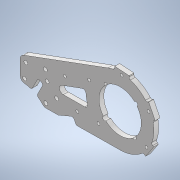
# Autodesk Inventor part: motor_h_6
Saved by Autodesk Inventor 2020 (Build 240168000, 168)
## iProperties
Created: 2020-11-16
Part Number: motor_h_6
Material: Generic
Document SubType Name: Modeling
Designer: Shuang Peng
Density: 1 g/cm^3
Appearance: Default
Author: Shuang Peng
Autodesk Inventor part; units mm, degrees
ref_plane "YZ Plane" through (0, 0, 0) normal (1, 0, 0) x (0, 1, 0)
ref_plane "XZ Plane" through (0, 0, 0) normal (0, 1, 0) x (-1, 0, 0)
ref_plane "XY Plane" through (0, 0, 0) normal (0, 0, 1) x (1, 0, 0)
sketch "Sketch1" plane through (0, 0, 0) normal (0, 0, 1) x (1, 0, 0)
  circle A0 centre (0.5323, 0.2768) radius 22 projected
  circle A1 centre (0.5323, 0.2768) radius 35
  line L0 (-78.3162, -45.1599) -> (-53.6214, -37.0254) projected
  line L1 (-86.2398, -25.4424) -> (-79.6785, -13.735) projected
  line L2 (-88.6848, -24.2091) -> (-83.1688, -11.9743) projected
  line L3 (-114.2243, 0.9226) -> (-109.1572, -20.6268) projected
  circle A2 centre (-76.7687, -31.0745) radius 2 projected
  circle A3 centre (-65.488, -21.1879) radius 2 projected
  circle A4 centre (-98.8432, -19.9393) radius 2 projected
  circle A5 centre (-97.5964, -4.9912) radius 2 projected
  line L4 (-9.6196, 33.6521) -> (-104.4582, 6.5421) projected
  line L5 (-65.488, -21.1879) -> (-97.5964, -4.9912)
  line L6 (-97.5964, -4.9912) -> (-98.8432, -19.9393)
  line L7 (-98.8432, -19.9393) -> (-76.7687, -31.0745)
  line L8 (-76.7687, -31.0745) -> (-65.488, -21.1879)
  arc A6 (-123.4396, -70.4026) -> (-119.9166, -61.7947) centre (-170.0752, -46.291) ccw projected
  arc A7 (-116.2774, -61.379) -> (-119.9166, -61.7947) centre (-118.0058, -62.3853) ccw projected
  arc A8 (-116.2774, -61.379) -> (-113.2569, -65.1861) centre (-101.5862, -52.8251) ccw projected
  arc A9 (-113.5219, -68.3053) -> (-113.2569, -65.1861) centre (-114.63, -66.6404) ccw projected
  line L9 (-113.5219, -68.3053) -> (-120.5549, -72.9861) projected
  arc A10 (-123.4396, -70.4026) -> (-120.5549, -72.9861) centre (-121.663, -71.3211) ccw projected
  arc A11 (-108.797, -37.4302) -> (-114.395, -41.6477) centre (-101.5862, -52.8251) ccw projected
  arc A12 (-117.8899, -40.5514) -> (-114.395, -41.6477) centre (-115.9019, -40.3327) ccw projected
  arc A13 (-117.8899, -40.5514) -> (-120.2217, -29.8328) centre (-170.0752, -46.291) ccw projected
  arc A14 (-117.1337, -27.5974) -> (-120.2217, -29.8328) centre (-118.3225, -29.2058) ccw projected
  line L10 (-117.1337, -27.5974) -> (-108.4566, -34.0106) projected
  arc A15 (-108.797, -37.4302) -> (-108.4566, -34.0106) centre (-109.6453, -35.619) ccw projected
  circle A16 centre (-99.5268, -40.1525) radius 2.05 projected
  circle A17 centre (-114.2588, -50.7657) radius 2.05 projected
  circle A18 centre (-103.6456, -65.4977) radius 2.05 projected
  circle A19 centre (-88.9136, -54.8845) radius 2.05 projected
  circle A20 centre (-108.8928, -42.6829) radius 1.55 projected
  circle A21 centre (-94.2796, -62.9673) radius 1.55 projected
  circle A22 centre (-111.7284, -60.1317) radius 1.55 projected
  circle A23 centre (-91.444, -45.5185) radius 1.55 projected
  line L11 (-163.6957, -101.6981) -> (-176.5687, -110.2656) projected
  arc A24 (-179.6679, -108.4127) -> (-176.5687, -110.2656) centre (-177.6768, -108.6006) ccw projected
  arc A25 (-179.6679, -108.4127) -> (-179.6132, -104.4918) centre (-204.0596, -106.1116) ccw projected
  arc A26 (-178.2819, -101.796) -> (-179.6132, -104.4918) centre (-176.6198, -104.2934) ccw projected
  line L12 (-178.2819, -101.796) -> (-174.2482, -99.1114) projected
  arc A27 (-171.3549, -98.2753) -> (-174.2482, -99.1114) centre (-171.4779, -103.2738) ccw projected
  arc A28 (-171.3549, -98.2753) -> (-164.9991, -98.0427) centre (-170.0752, -46.291) ccw projected
  arc A29 (-163.6957, -101.6981) -> (-164.9991, -98.0427) centre (-164.8038, -100.0331) ccw projected
  arc A30 (-215.7892, -71.0747) -> (-212.0199, -77.0261) centre (-170.0752, -46.291) ccw projected
  arc A31 (-212.9841, -80.1) -> (-212.0199, -77.0261) centre (-213.6331, -78.2082) ccw projected
  arc A32 (-212.9841, -80.1) -> (-217.4538, -82.094) centre (-204.0596, -106.1116) ccw projected
  arc A33 (-220.4168, -80.1368) -> (-217.4538, -82.094) centre (-218.4279, -80.3472) ccw projected
  line L13 (-220.4168, -80.1368) -> (-219.5364, -71.8174) projected
  arc A34 (-215.7892, -71.0747) -> (-219.5364, -71.8174) centre (-217.5475, -72.0279) ccw projected
  circle A35 centre (-195.3093, -126.2965) radius 2.05 projected
  circle A36 centre (-183.8747, -97.3613) radius 2.05 projected
  circle A37 centre (-212.81, -85.9267) radius 2.05 projected
  circle A38 centre (-224.2445, -114.862) radius 2.05 projected
  circle A39 centre (-156.8228, -41.9256) radius 2.1 projected
  circle A40 centre (-142.9852, -15.9584) radius 2.1 projected
  circle A41 centre (-167.2295, -32.6314) radius 2.1 projected
  circle A42 centre (-182.799, -7.6641) radius 2.1 projected
  circle A43 centre (-180.482, -36.9968) radius 2.1 projected
  circle A44 centre (-209.889, -37.9967) radius 2.1 projected
  circle A45 centre (-183.3277, -50.6564) radius 2.1 projected
  circle A46 centre (-197.1652, -76.6237) radius 2.1 projected
  circle A47 centre (-172.9209, -59.9507) radius 2.1 projected
  circle A48 centre (-157.3514, -84.918) radius 2.1 projected
  circle A49 centre (-130.2614, -54.5854) radius 2.1 projected
  circle A50 centre (-159.6685, -55.5853) radius 2.1 projected
  line L14 (-151.4769, -35.1571) -> (-159.0568, -36.2537) projected
  arc A51 (-161.3422, -34.2126) -> (-159.0568, -36.2537) centre (-159.3431, -34.2743) ccw projected
  line L15 (-161.3422, -34.2126) -> (-161.1059, -26.5575) projected
  arc A52 (-156.5463, -24.0882) -> (-161.1059, -26.5575) centre (-158.1073, -26.65) ccw projected
  arc A53 (-149.5366, -30.3485) -> (-156.5463, -24.0882) centre (-170.0752, -46.291) ccw projected
  arc A54 (-151.4769, -35.1571) -> (-149.5366, -30.3485) centre (-151.9064, -32.188) ccw projected
  line L16 (-170.4183, -24.6174) -> (-173.2586, -31.7301) projected
  arc A55 (-176.1689, -32.6888) -> (-173.2586, -31.7301) centre (-175.1159, -30.9884) ccw projected
  line L17 (-176.1689, -32.6888) -> (-182.6803, -28.6566) projected
  arc A56 (-182.539, -23.4732) -> (-182.6803, -28.6566) centre (-181.1009, -26.106) ccw projected
  arc A57 (-173.6125, -20.5328) -> (-182.539, -23.4732) centre (-170.0752, -46.291) ccw projected
  arc A58 (-170.4183, -24.6174) -> (-173.6125, -20.5328) centre (-173.2044, -23.5049) ccw projected
  line L18 (-189.0166, -35.7513) -> (-184.277, -41.7674) projected
  arc A59 (-184.9019, -44.7672) -> (-184.277, -41.7674) centre (-185.848, -43.0051) ccw projected
  line L19 (-184.9019, -44.7672) -> (-191.6497, -48.3902) projected
  arc A60 (-196.0679, -45.6761) -> (-191.6497, -48.3902) centre (-193.0688, -45.747) ccw projected
  arc A61 (-194.1512, -36.4753) -> (-196.0679, -45.6761) centre (-170.0752, -46.291) ccw projected
  arc A62 (-189.0166, -35.7513) -> (-194.1512, -36.4753) centre (-191.3732, -37.6079) ccw projected
  line L20 (-188.6736, -57.4249) -> (-181.0937, -56.3283) projected
  arc A63 (-178.8083, -58.3694) -> (-181.0937, -56.3283) centre (-180.8073, -58.3077) ccw projected
  line L21 (-178.8083, -58.3694) -> (-179.0445, -66.0246) projected
  arc A64 (-183.6042, -68.4939) -> (-179.0445, -66.0246) centre (-182.0431, -65.932) ccw projected
  arc A65 (-190.6139, -62.2336) -> (-183.6042, -68.4939) centre (-170.0752, -46.291) ccw projected
  arc A66 (-188.6736, -57.4249) -> (-190.6139, -62.2336) centre (-188.244, -60.394) ccw projected
  line L22 (-169.7321, -67.9646) -> (-166.8919, -60.8519) projected
  arc A67 (-163.9815, -59.8933) -> (-166.8919, -60.8519) centre (-165.0345, -61.5936) ccw projected
  line L23 (-163.9815, -59.8933) -> (-157.4701, -63.9255) projected
  arc A68 (-157.6114, -69.1089) -> (-157.4701, -63.9255) centre (-159.0496, -66.4761) ccw projected
  arc A69 (-166.5379, -72.0493) -> (-157.6114, -69.1089) centre (-170.0752, -46.291) ccw projected
  arc A70 (-169.7321, -67.9646) -> (-166.5379, -72.0493) centre (-166.9461, -69.0772) ccw projected
  line L24 (-151.1338, -56.8307) -> (-155.8734, -50.8146) projected
  arc A71 (-155.2485, -47.8149) -> (-155.8734, -50.8146) centre (-154.3024, -49.5769) ccw projected
  line L25 (-155.2485, -47.8149) -> (-148.5008, -44.1919) projected
  arc A72 (-144.0825, -46.906) -> (-148.5008, -44.1919) centre (-147.0817, -46.835) ccw projected
  arc A73 (-145.9993, -56.1068) -> (-144.0825, -46.906) centre (-170.0752, -46.291) ccw projected
  arc A74 (-151.1338, -56.8307) -> (-145.9993, -56.1068) centre (-148.7773, -54.9742) ccw projected
  arc A75 (-216.0243, -48.4556) -> (-208.3152, -71.8586) centre (-170.0752, -46.291) ccw projected
  arc A76 (-211.8355, -44.272) -> (-216.0243, -48.4556) centre (-212.0287, -48.2673) ccw projected
  line L26 (-211.8355, -44.272) -> (-205.407, -44.5828) projected
  arc A77 (-202.5538, -47.4705) -> (-205.407, -44.5828) centre (-205.5518, -47.5793) ccw projected
  arc A78 (-202.5538, -47.4705) -> (-196.8964, -64.6451) centre (-170.0752, -46.291) ccw projected
  arc A79 (-197.4748, -68.6631) -> (-196.8964, -64.6451) centre (-199.3722, -66.3394) ccw projected
  line L27 (-197.4748, -68.6631) -> (-202.4602, -72.7337) projected
  arc A80 (-208.3152, -71.8586) -> (-202.4602, -72.7337) centre (-204.99, -69.6353) ccw projected
  arc A81 (-191.1752, -87.1663) -> (-167.0531, -92.1917) centre (-170.0752, -46.291) ccw projected
  arc A82 (-192.7039, -81.447) -> (-191.1752, -87.1663) centre (-189.3404, -83.612) ccw projected
  line L28 (-192.7039, -81.447) -> (-189.2204, -76.0351) projected
  arc A83 (-185.2931, -75.008) -> (-189.2204, -76.0351) centre (-186.6978, -77.6588) ccw projected
  arc A84 (-185.2931, -75.008) -> (-167.5907, -78.6959) centre (-170.0752, -46.291) ccw projected
  arc A85 (-164.4002, -81.2059) -> (-167.5907, -78.6959) centre (-167.3614, -81.6872) ccw projected
  line L29 (-164.4002, -81.2059) -> (-163.3677, -87.5586) projected
  arc A86 (-167.0531, -92.1917) -> (-163.3677, -87.5586) centre (-167.3159, -88.2003) ccw projected
  arc A87 (-145.2262, -85.0018) -> (-128.813, -66.6241) centre (-170.0752, -46.291) ccw projected
  arc A88 (-150.9436, -83.466) -> (-145.2262, -85.0018) centre (-147.3869, -81.6357) ccw projected
  line L30 (-150.9436, -83.466) -> (-153.8887, -77.7433) projected
  arc A89 (-152.8145, -73.8286) -> (-153.8887, -77.7433) centre (-151.2212, -76.3705) ccw projected
  arc A90 (-152.8145, -73.8286) -> (-140.7695, -60.3418) centre (-170.0752, -46.291) ccw projected
  arc A91 (-137.0006, -58.8338) -> (-140.7695, -60.3418) centre (-138.0644, -61.6388) ccw projected
  line L31 (-137.0006, -58.8338) -> (-130.9827, -61.1159) projected
  arc A92 (-128.813, -66.6241) -> (-130.9827, -61.1159) centre (-132.4011, -64.856) ccw projected
  arc A93 (-124.1262, -44.1265) -> (-131.8352, -20.7235) centre (-170.0752, -46.291) ccw projected
  arc A94 (-128.3149, -48.3101) -> (-124.1262, -44.1265) centre (-128.1217, -44.3147) ccw projected
  line L32 (-128.3149, -48.3101) -> (-134.7435, -47.9993) projected
  arc A95 (-137.5966, -45.1116) -> (-134.7435, -47.9993) centre (-134.5986, -45.0028) ccw projected
  arc A96 (-137.5966, -45.1116) -> (-143.254, -27.9369) centre (-170.0752, -46.291) ccw projected
  arc A97 (-142.6756, -23.9189) -> (-143.254, -27.9369) centre (-140.7782, -26.2427) ccw projected
  line L33 (-142.6756, -23.9189) -> (-137.6903, -19.8484) projected
  arc A98 (-131.8352, -20.7235) -> (-137.6903, -19.8484) centre (-135.1604, -22.9467) ccw projected
  arc A99 (-148.9752, -5.4157) -> (-173.0974, -0.3904) centre (-170.0752, -46.291) ccw projected
  arc A100 (-147.4465, -11.1351) -> (-148.9752, -5.4157) centre (-150.81, -8.9701) ccw projected
  line L34 (-147.4465, -11.1351) -> (-150.93, -16.547) projected
  arc A101 (-154.8573, -17.574) -> (-150.93, -16.547) centre (-153.4526, -14.9232) ccw projected
  arc A102 (-154.8573, -17.574) -> (-172.5597, -13.8861) centre (-170.0752, -46.291) ccw projected
  arc A103 (-175.7502, -11.3762) -> (-172.5597, -13.8861) centre (-172.7891, -10.8949) ccw projected
  line L35 (-175.7502, -11.3762) -> (-176.7828, -5.0235) projected
  arc A104 (-173.0974, -0.3904) -> (-176.7828, -5.0235) centre (-172.8346, -4.3818) ccw projected
  arc A105 (-194.9243, -7.5803) -> (-211.3374, -25.958) centre (-170.0752, -46.291) ccw projected
  arc A106 (-189.2068, -9.116) -> (-194.9243, -7.5803) centre (-192.7635, -10.9464) ccw projected
  line L36 (-189.2068, -9.116) -> (-186.2617, -14.8387) projected
  arc A107 (-187.3359, -18.7535) -> (-186.2617, -14.8387) centre (-188.9292, -16.2115) ccw projected
  arc A108 (-187.3359, -18.7535) -> (-199.3809, -32.2402) centre (-170.0752, -46.291) ccw projected
  arc A109 (-203.1498, -33.7483) -> (-199.3809, -32.2402) centre (-202.0861, -30.9432) ccw projected
  line L37 (-203.1498, -33.7483) -> (-209.1677, -31.4662) projected
  arc A110 (-211.3374, -25.958) -> (-209.1677, -31.4662) centre (-207.7494, -27.7261) ccw projected
  circle A111 centre (-204.0596, -106.1116) radius 16 projected
  circle A112 centre (-170.0752, -46.291) radius 8 projected
  circle A113 centre (-101.5862, -52.8251) radius 8 projected
  circle A114 centre (-214.7177, -133.082) radius 1.5 projected
  circle A115 centre (-219.3611, -19.837) radius 1.5 projected
  circle A116 centre (-193.5118, 4.9009) radius 1.5 projected
  circle A117 centre (-78.1429, -40.8914) radius 1.5 projected
  circle A118 centre (-111.8739, -77.0359) radius 1.5 projected
  circle A119 centre (-81.5873, -69.9144) radius 1.5 projected
  circle A120 centre (-105.9215, -26.8789) radius 1.5 projected
  circle A121 centre (-174.6475, 9.4585) radius 1.5 projected
  circle A122 centre (-207.6497, -4.3619) radius 1.5 projected
  circle A123 centre (-232.6899, -112.2194) radius 1.5 projected
  circle A124 centre (-187.3388, -130.1411) radius 1.5 projected
  line L38 (-182.2334, -121.243) -> (-118.1865, -78.6172) projected
  arc A125 (-116.0255, -78.5818) -> (-118.1865, -78.6172) centre (-117.0784, -80.2822) ccw projected
  line L39 (-116.0255, -78.5818) -> (-110.3159, -82.1175) projected
  line L40 (-110.3159, -82.1175) -> (-109.1162, -80.1802) projected
  arc A126 (-107.0138, -79.274) -> (-109.1162, -80.1802) centre (-107.4158, -81.2331) ccw projected
  arc A127 (-107.0138, -79.274) -> (-84.9408, -74.0838) centre (-101.5862, -52.8251) ccw projected
  arc A128 (-82.6548, -73.9581) -> (-84.9408, -74.0838) centre (-83.7078, -75.6585) ccw projected
  line L41 (-82.6548, -73.9581) -> (-80.7175, -75.1578) projected
  line L42 (-80.7175, -75.1578) -> (-76.5057, -68.3563) projected
  line L43 (-76.5057, -68.3563) -> (-80.8261, -65.6809) projected
  arc A129 (-81.5538, -63.0698) -> (-80.8261, -65.6809) centre (-79.7732, -63.9805) ccw projected
  arc A130 (-81.5538, -63.0698) -> (-79.7124, -47.5537) centre (-101.5862, -52.8251) ccw projected
  arc A131 (-78.3938, -45.1855) -> (-79.7124, -47.5537) centre (-77.7681, -47.0851) ccw projected
  line L44 (-78.3938, -45.1855) -> (-73.5672, -43.5956) projected
  line L45 (-73.5672, -43.5956) -> (-76.0701, -35.9972) projected
  line L46 (-76.0701, -35.9972) -> (-78.2344, -36.7101) projected
  arc A132 (-80.4274, -36.0529) -> (-78.2344, -36.7101) centre (-78.8601, -34.8105) ccw projected
  arc A133 (-80.4274, -36.0529) -> (-100.6725, -25.8406) centre (-101.5862, -52.8251) ccw projected
  arc A134 (-102.5044, -24.4675) -> (-100.6725, -25.8406) centre (-100.6048, -23.8417) ccw projected
  line L47 (-102.5044, -24.4675) -> (-103.2174, -22.3032) projected
  line L48 (-103.2174, -22.3032) -> (-109.8332, -24.4825) projected
  arc A135 (-111.6477, -24.1912) -> (-109.8332, -24.4825) centre (-110.4589, -22.5829) ccw projected
  line L49 (-111.6477, -24.1912) -> (-138.8709, -4.0709) projected
  arc A136 (-138.8709, -4.0709) -> (-157.489, 4.6779) centre (-170.0752, -46.291) ccw projected
  arc A137 (-158.9675, 7.0275) -> (-157.489, 4.6779) centre (-157.0095, 6.6196) ccw projected
  line L50 (-158.9675, 7.0275) -> (-157.9255, 12.0294) projected
  line L51 (-157.9255, 12.0294) -> (-173.905, 13.0221) projected
  arc A138 (-173.905, 13.0221) -> (-179.0599, 12.4626) centre (-170.0752, -46.291) ccw projected
  line L52 (-179.0599, 12.4626) -> (-178.9132, 11.5029) projected
  arc A139 (-180.5204, 9.2351) -> (-178.9132, 11.5029) centre (-180.8902, 11.2006) ccw projected
  arc A140 (-180.5204, 9.2351) -> (-188.9488, 6.9634) centre (-170.0752, -46.291) ccw projected
  arc A141 (-191.4781, 8.1164) -> (-188.9488, 6.9634) centre (-189.6169, 8.8485) ccw projected
  line L53 (-191.4781, 8.1164) -> (-191.9672, 9.3596) projected
  arc A142 (-191.9672, 9.3596) -> (-197.6643, 6.7664) centre (-170.0752, -46.291) ccw projected
  line L54 (-197.6643, 6.7664) -> (-207.7018, 0.19) projected
  arc A143 (-207.7018, 0.19) -> (-212.3543, -3.9976) centre (-170.0752, -46.291) ccw projected
  line L55 (-212.3543, -3.9976) -> (-211.4098, -4.9425) projected
  arc A144 (-211.3627, -7.7217) -> (-211.4098, -4.9425) centre (-212.8242, -6.3564) ccw projected
  arc A145 (-211.3627, -7.7217) -> (-216.811, -14.5418) centre (-170.0752, -46.291) ccw projected
  arc A146 (-219.5321, -15.1098) -> (-216.811, -14.5418) centre (-218.4654, -13.418) ccw projected
  line L56 (-219.5321, -15.1098) -> (-220.3533, -14.592) projected
  arc A147 (-220.3533, -14.592) -> (-222.9247, -19.0947) centre (-170.0752, -46.291) ccw projected
  line L57 (-222.9247, -19.0947) -> (-228.3956, -34.1413) projected
  line L58 (-228.3956, -34.1413) -> (-223.3938, -35.1833) projected
  arc A148 (-221.8301, -37.477) -> (-223.3938, -35.1833) centre (-223.8017, -37.1413) ccw projected
  arc A149 (-221.8301, -37.477) -> (-222.2837, -40.7658) centre (-170.0752, -46.291) ccw projected
  line L59 (-222.2837, -40.7658) -> (-228.8679, -102.9811) projected
  arc A150 (-234.3963, -108.3336) -> (-228.8679, -102.9811) centre (-234.8346, -102.3497) ccw projected
  line L60 (-234.3963, -108.3336) -> (-236.9714, -108.5222) projected
  line L61 (-236.9714, -108.5222) -> (-236.5332, -114.5062) projected
  line L62 (-236.5332, -114.5062) -> (-234.3924, -116.3548) projected
  line L63 (-234.3924, -116.3548) -> (-232.2123, -116.1951) projected
  arc A151 (-230.2297, -117.3977) -> (-232.2123, -116.1951) centre (-232.0662, -118.1897) ccw projected
  arc A152 (-230.2297, -117.3977) -> (-219.5435, -130.0386) centre (-204.0596, -106.1116) ccw projected
  arc A153 (-218.77, -132.4527) -> (-219.5435, -130.0386) centre (-220.6301, -131.7177) ccw projected
  line L64 (-218.77, -132.4527) -> (-219.1728, -133.472) projected
  line L65 (-219.1728, -133.472) -> (-218.0478, -136.0671) projected
  line L66 (-218.0478, -136.0671) -> (-214.3278, -137.5372) projected
  line L67 (-214.3278, -137.5372) -> (-211.7327, -136.4122) projected
  line L68 (-211.7327, -136.4122) -> (-211.3299, -135.3929) projected
  arc A154 (-209.1151, -134.1596) -> (-211.3299, -135.3929) centre (-209.4699, -136.1279) ccw projected
  arc A155 (-209.1151, -134.1596) -> (-192.6744, -132.2387) centre (-204.0596, -106.1116) ccw projected
  arc A156 (-190.4053, -132.7163) -> (-192.6744, -132.2387) centre (-191.8754, -134.0722) ccw projected
  line L69 (-190.4053, -132.7163) -> (-188.9233, -134.3231) projected
  line L70 (-188.9233, -134.3231) -> (-186.0971, -134.4374) projected
  line L71 (-186.0971, -134.4374) -> (-181.6866, -130.3696) projected
  line L72 (-181.6866, -130.3696) -> (-183.1386, -128.7953) projected
  arc A157 (-182.2334, -121.243) -> (-183.1386, -128.7953) centre (-179.4631, -125.4054) ccw projected
  circle A158 centre (-98.8432, -19.9393) radius 4.5
  circle A159 centre (-76.7687, -31.0745) radius 4.5
  circle A160 centre (-101.5862, -52.8251) radius 28.5
  circle A161 centre (-97.5964, -4.9912) radius 6
  circle A162 centre (-65.488, -21.1879) radius 6
  arc A163 (33.1414, -11.2539) -> (34.2988, 6.971) centre (0, 0) ccw projected
  line L73 (-98.8432, -19.9393) -> (-103.3426, -20.0156)
  line L74 (-97.5964, -4.9912) -> (-103.5955, -5.0929)
  line L75 (-103.5955, -5.0929) -> (-103.3426, -20.0156)
  line L76 (0, 0) -> (0.3834, -34.7229)
  line L77 (0.3834, -34.7229) -> (-76.719, -35.5742)
  line L78 (0, 0) -> (-12.1292, 32.9063)
  line L79 (-12.1292, 32.9063) -> (-99.6715, 0.6385)
  line L80 (-99.6715, 0.6385) -> (-97.5964, -4.9912)
  point P0 (0, 0)
  point P1 (-99.2173, -24.4238)
  point P2 (-80.1529, -34.0405)
  dimension "d1" = 9
  dimension "d2" = 9
  dimension "d0" = 70
  dimension "d3" = 12
  dimension "d4" = 12
  constraints: 24 end point, 6 coincident, 5 perpendicular, 4 centre point, 4 point on circle, 1 parallel, 8 other
  measures "d0" diameter of A1
  measures "d3" diameter of A161
  measures "d4" diameter of A162
extrude "Extrusion1" add sketch "Sketch1" against normal blind 5 contours A0 L78 A1 L76 | A0 L76 A1 L78 | A1 L77 A159 L8 A162 L5 A161 L79 | L80 A5 L74 A161 | A161 L5 A5 L80 | A159 L7 A2 L8 | L74 A5 L6 A161 | A161 L6 A158 L75 | A160 A158 L7 A159 | A161 L6 A5 L5 | L5 A162 L8 A159 L7 A158 L6 A161 | L73 A4 L7 A158 | A158 L6 A4 L73 | L8 A2 L7 A159 | A158 L7 A4 L6 | A162 L5 A3 L8 | L8 A3 L5 A162
sketch "Sketch2" plane through (0, 0, 0) normal (0, 0, 1) x (1, 0, 0)
  line L0 (-86.2398, -25.4424) -> (-79.6785, -13.735) projected
  line L1 (-88.6848, -24.2091) -> (-83.1688, -11.9743) projected
  line L2 (-79.6785, -13.735) -> (-83.1688, -11.9743)
  line L3 (-88.6848, -24.2091) -> (-86.2398, -25.4424)
  line L4 (-81.4237, -12.8547) -> (-87.4623, -24.8257)
  line L5 (-81.4237, -12.8547) -> (-85.4771, -20.8902)
  line L6 (-78.52, -13.7594) -> (-83.877, -11.0571)
  line L7 (-83.877, -11.0571) -> (-92.4342, -28.021)
  line L8 (-92.4342, -28.021) -> (-87.0772, -30.7233)
  line L9 (-87.0772, -30.7233) -> (-78.52, -13.7594)
  line L10 (-78.52, -13.7594) -> (-92.4342, -28.021) construction
  line L11 (-83.877, -11.0571) -> (-87.0772, -30.7233) construction
  point P0 (0, 0)
  dimension "d7" = 9
  dimension "d8" = 6
  dimension "d9" = 19
  constraints: 20 end point, 4 midpoint, 3 parallel, 3 perpendicular, 1 point on line
  measures "d7" distance of L4.start L5.end
  measures "d8" distance of L6.start L6.end
  measures "d9" distance of L7.end L6.end
extrude "Extrusion2" cut sketch "Sketch2" against normal blind 5 contours L3 L4 L2 L0 | L3 L1 L2 L4 | L9 L8 L7 L6
fillet "Fillet1" radius 2 4 edges at (-86.1432, -28.8718, -2.5) (-91.5002, -26.1695, -2.5) (-83.877, -11.0571, -2.5) (-78.52, -13.7594, -2.5)
thicken "Thicken1" operation add thickness 2 both sides no extend neighbours yes toward (-0.4503786, -0.8928377, 0) faces at (-80.9009, -12.5584, -1.6667)
sketch "Sketch3" plane through (0, 0, 0) normal (0, 0, 1) x (1, 0, 0)
  line L0 (-49.3684, -35.6245) -> (-70.3559, -42.5378) projected
  line L1 (-71.1917, -39.7779) -> (-50.8496, -31.0458) projected
  line L2 (-90.714, -24.6109) -> (-85.6785, -14.6284) projected
  arc A0 (-82.9921, -13.7435) -> (-85.6785, -14.6284) centre (-83.8929, -15.5292) ccw projected
  line L3 (-82.9921, -13.7435) -> (-81.2064, -14.6443) projected
  arc A1 (-80.3215, -17.3307) -> (-81.2064, -14.6443) centre (-82.1072, -16.43) ccw projected
  line L4 (-80.3215, -17.3307) -> (-85.357, -27.3131) projected
  arc A2 (-85.357, -27.3131) -> (-84.7526, -29.8277) centre (-83.5713, -28.2139) ccw projected
  arc A3 (-80.1529, -34.0405) -> (-84.7526, -29.8277) centre (-101.5862, -52.8251) ccw projected
  arc A4 (-80.1529, -34.0405) -> (-76.719, -35.5742) centre (-76.7687, -31.0745) ccw projected
  line L5 (-76.719, -35.5742) -> (0.3834, -34.7229) projected
  arc A5 (0.3834, -34.7229) -> (-12.1292, 32.9063) centre (0.5323, 0.2768) ccw projected
  line L6 (-12.1292, 32.9063) -> (-99.6715, 0.6385) projected
  arc A6 (-99.6715, 0.6385) -> (-103.5955, -5.0929) centre (-97.5964, -4.9912) ccw projected
  line L7 (-103.5955, -5.0929) -> (-103.3426, -20.0156) projected
  arc A7 (-103.3426, -20.0156) -> (-99.2173, -24.4238) centre (-98.8432, -19.9393) ccw projected
  arc A8 (-93.0955, -25.6193) -> (-99.2173, -24.4238) centre (-101.5862, -52.8251) ccw projected
  arc A9 (-93.0955, -25.6193) -> (-90.714, -24.6109) centre (-92.4997, -23.7101) ccw projected
  circle A10 centre (-98.8432, -19.9393) radius 2 projected
  circle A11 centre (-65.488, -21.1879) radius 2 projected
  circle A12 centre (-97.5964, -4.9912) radius 2 projected
  circle A13 centre (-76.7687, -31.0745) radius 2 projected
  line L8 (-76.719, -35.5742) -> (0.3834, -34.7229) projected
  line L9 (-76.719, -35.5742) -> (-63.7198, -35.4307)
  line L10 (-63.7198, -35.4307) -> (-48.0982, -28.7249)
  line L11 (-48.0982, -28.7249) -> (-45.307, -35.2274)
  point P0 (0, 0)
  point P1 (-63.7198, -35.4307)
  dimension "d15" = 13
  dimension "d16" = 17
  constraints: 6 end point, 2 point on line, 1 parallel, 1 perpendicular
  measures "d15" distance of L5.start L9.end
  measures "d16" distance of L9.end L10.end
extrude "Extrusion3" cut sketch "Sketch3" against normal blind 5 contours L5 L10 L11
sketch "Sketch5" plane through (0, 0, 0) normal (0, 0, 1) x (1, 0, 0)
  circle A0 centre (27.8919, -18.555) radius 1.5 projected
  circle A1 centre (30.0151, 14.8776) radius 1.5 projected
  circle A2 centre (2.1232, 33.4327) radius 1.5 projected
  point P0 (0, 0)
extrude "Extrusion5" cut sketch "Sketch5" against normal blind 5
fillet "Fillet2" radius 3 1 edges at (-48.0982, -28.7249, -2.5)
sketch "Sketch6" plane through (0, 0, 0) normal (0, 0, 1) x (1, 0, 0)
  circle A0 centre (-31.704, 12.2896) radius 2.1 projected
  circle A1 centre (-57.0448, 2.9708) radius 2.1 projected
  circle A2 centre (-22.0609, -22.1123) radius 2.1 projected
  circle A3 centre (-44.0603, -22.2767) radius 2.1 projected
  point P0 (0, 0)
hole "Hole1" at (-22.0609, -22.1123, 0) at (-44.0603, -22.2767, 0) at (-31.704, 12.2896, 0) at (-57.0448, 2.9708, 0) direction (0, 0, -1) diameter 3 end through all
fillet "Fillet3" radius 2 1 edges at (-45.307, -35.2274, -2.5)
sketch "Sketch8" plane through (0, 0, 0) normal (0, 0, 1) x (1, 0, 0)
  circle A0 centre (-31.704, 12.2896) radius 1.5 projected
  circle A1 centre (-22.0609, -22.1123) radius 1.5 projected
  circle A2 centre (-44.0603, -22.2767) radius 1.5 projected
  circle A3 centre (-57.0448, 2.9708) radius 1.5 projected
  circle A4 centre (2.1232, 33.4327) radius 1.5 projected
  circle A5 centre (30.0151, 14.8776) radius 1.5 projected
  circle A6 centre (27.8919, -18.555) radius 1.5 projected
  arc A7 (-45.8331, -34.0017) -> (-43.9732, -35.2127) centre (-43.9953, -33.2128) ccw projected
  line L0 (-43.9732, -35.2127) -> (0.3834, -34.7229) projected
  arc A8 (0.3834, -34.7229) -> (-12.1292, 32.9063) centre (0.5323, 0.2768) ccw projected
  line L1 (-12.1292, 32.9063) -> (-99.6715, 0.6385) projected
  arc A9 (-99.6715, 0.6385) -> (-103.5955, -5.0929) centre (-97.5964, -4.9912) ccw projected
  line L2 (-103.5955, -5.0929) -> (-103.3426, -20.0156) projected
  arc A10 (-103.3426, -20.0156) -> (-99.2173, -24.4238) centre (-98.8432, -19.9393) ccw projected
  arc A11 (-93.0955, -25.6193) -> (-99.2173, -24.4238) centre (-101.5862, -52.8251) ccw projected
  arc A12 (-93.0955, -25.6193) -> (-90.714, -24.6109) centre (-92.4997, -23.7101) ccw projected
  line L3 (-90.714, -24.6109) -> (-85.6785, -14.6284) projected
  arc A13 (-82.9921, -13.7435) -> (-85.6785, -14.6284) centre (-83.8929, -15.5292) ccw projected
  line L4 (-82.9921, -13.7435) -> (-81.2064, -14.6443) projected
  arc A14 (-80.3215, -17.3307) -> (-81.2064, -14.6443) centre (-82.1072, -16.43) ccw projected
  line L5 (-80.3215, -17.3307) -> (-85.357, -27.3131) projected
  arc A15 (-85.357, -27.3131) -> (-84.7526, -29.8277) centre (-83.5713, -28.2139) ccw projected
  arc A16 (-80.1529, -34.0405) -> (-84.7526, -29.8277) centre (-101.5862, -52.8251) ccw projected
  arc A17 (-80.1529, -34.0405) -> (-76.719, -35.5742) centre (-76.7687, -31.0745) ccw projected
  line L6 (-76.719, -35.5742) -> (-63.7198, -35.4307) projected
  line L7 (-63.7198, -35.4307) -> (-50.855, -29.9083) projected
  arc A18 (-46.9148, -31.4817) -> (-50.855, -29.9083) centre (-49.6716, -32.6651) ccw projected
  line L8 (-46.9148, -31.4817) -> (-45.8331, -34.0017) projected
  circle A19 centre (-98.8432, -19.9393) radius 2 projected
  circle A20 centre (-65.488, -21.1879) radius 2 projected
  circle A21 centre (-97.5964, -4.9912) radius 2 projected
  circle A22 centre (-76.7687, -31.0745) radius 2 projected
  line L9 (-98.8432, -19.9393) -> (0, 0)
  circle A23 centre (0, 0) radius 35
  line L10 (-31.704, 12.2896) -> (-57.0448, 2.9708)
  line L11 (-44.0603, -22.2767) -> (-22.0609, -22.1123)
  line L12 (-29.6578, 4.5183) -> (-59.9756, -6.6307)
  line L13 (-26.456, -14.1449) -> (-58.5651, -14.3848)
  circle A24 centre (0, 0) radius 30
  arc A25 (-59.9756, -6.6307) -> (-58.5651, -14.3848) centre (-58.595, -10.3849) ccw
  point P0 (-31.9961, -14.1863)
  point P1 (-34.9041, 2.589)
  dimension "d39" = 70
  dimension "d40" = 8
  dimension "d41" = 8
  dimension "d43" = 4
  constraints: 10 end point, 4 point on circle, 3 centre point, 2 coincident, 2 parallel, 2 tangent
  measures "d39" diameter of A23
  measures "d40" distance between parallel lines of L11 L13
  measures "d41" distance between parallel lines of L10 L12
  measures "d43" radius of A25
extrude "Extrusion7" cut sketch "Sketch8" against normal blind 10 contours A23 L9 A25 L12 | A23 L13 A25 L9
fillet "Fillet4" radius 3 2 edges at (-31.9961, -14.1863, -2.5) (-34.9041, 2.589, -2.5)
sketch "Sketch9" plane through (0, 0, -5) normal (0, 0, -1) x (-1, 0, 0)
  arc A0 (33.44, -10.3327) -> (34.9637, -1.5947) centre (0, 0) ccw projected
  arc A1 (38.996, 1.0843) -> (34.9637, -1.5947) centre (37.9605, -1.7314) ccw projected
  line L0 (38.996, 1.0843) -> (59.9756, -6.6307) projected
  arc A2 (58.5651, -14.3848) -> (59.9756, -6.6307) centre (58.595, -10.3849) ccw projected
  line L1 (58.5651, -14.3848) -> (36.2839, -14.2183) projected
  arc A3 (33.44, -10.3327) -> (36.2839, -14.2183) centre (36.3063, -11.2184) ccw projected
  arc A4 (43.9732, -35.2127) -> (45.8331, -34.0017) centre (43.9953, -33.2128) ccw projected
  line L2 (45.8331, -34.0017) -> (46.9148, -31.4817) projected
  arc A5 (50.855, -29.9083) -> (46.9148, -31.4817) centre (49.6716, -32.6651) ccw projected
  line L3 (50.855, -29.9083) -> (63.7198, -35.4307) projected
  line L4 (63.7198, -35.4307) -> (76.719, -35.5742) projected
  arc A6 (76.719, -35.5742) -> (80.1529, -34.0405) centre (76.7687, -31.0745) ccw projected
  arc A7 (84.7526, -29.8277) -> (80.1529, -34.0405) centre (101.5862, -52.8251) ccw projected
  arc A8 (84.7526, -29.8277) -> (85.357, -27.3131) centre (83.5713, -28.2139) ccw projected
  line L5 (85.357, -27.3131) -> (80.3215, -17.3307) projected
  arc A9 (81.2064, -14.6443) -> (80.3215, -17.3307) centre (82.1072, -16.43) ccw projected
  line L6 (81.2064, -14.6443) -> (82.9921, -13.7435) projected
  arc A10 (85.6785, -14.6284) -> (82.9921, -13.7435) centre (83.8929, -15.5292) ccw projected
  line L7 (85.6785, -14.6284) -> (90.714, -24.6109) projected
  arc A11 (90.714, -24.6109) -> (93.0955, -25.6193) centre (92.4997, -23.7101) ccw projected
  arc A12 (99.2173, -24.4238) -> (93.0955, -25.6193) centre (101.5862, -52.8251) ccw projected
  arc A13 (99.2173, -24.4238) -> (103.3426, -20.0156) centre (98.8432, -19.9393) ccw projected
  line L8 (103.3426, -20.0156) -> (103.5955, -5.0929) projected
  arc A14 (103.5955, -5.0929) -> (99.6715, 0.6385) centre (97.5964, -4.9912) ccw projected
  line L9 (99.6715, 0.6385) -> (12.1292, 32.9063) projected
  arc A15 (12.1292, 32.9063) -> (-0.3834, -34.7229) centre (-0.5323, 0.2768) ccw projected
  line L10 (-0.3834, -34.7229) -> (43.9732, -35.2127) projected
  circle A16 centre (31.704, 12.2896) radius 1.5 projected
  circle A17 centre (22.0609, -22.1123) radius 1.5 projected
  circle A18 centre (44.0603, -22.2767) radius 1.5 projected
  circle A19 centre (57.0448, 2.9708) radius 1.5 projected
  circle A20 centre (-2.1232, 33.4327) radius 1.5 projected
  circle A21 centre (-30.0151, 14.8776) radius 1.5 projected
  circle A22 centre (-27.8919, -18.555) radius 1.5 projected
  circle A23 centre (98.8432, -19.9393) radius 2 projected
  circle A24 centre (65.488, -21.1879) radius 2 projected
  circle A25 centre (97.5964, -4.9912) radius 2 projected
  circle A26 centre (76.7687, -31.0745) radius 2 projected
  line L11 (57.0448, 2.9708) -> (97.5964, -4.9912)
  circle A27 centre (77.3206, -1.0102) radius 2
  line L12 (77.3206, -1.0102) -> (75.394, -10.8229)
  circle A28 centre (75.394, -10.8229) radius 2
  dimension "d47" = 4
  dimension "d48" = 10
  dimension "d49" = 4
  constraints: 4 end point, 2 centre point, 1 coincident, 1 midpoint, 1 perpendicular
  measures "d47" diameter of A27
  measures "d48" distance of L12.start L12.end
  measures "d49" diameter of A28
extrude "Extrusion8" cut sketch "Sketch9" against normal blind 10 contours A27 L11 | L11 L12 A27 | L11 A27 L12 | A28
sketch "Sketch13" plane through (0, 0, 0) normal (0, 0, 1) x (1, 0, 0)
  circle A0 centre (-194.7129, -37.0724) radius 1.5 projected
  circle A1 centre (-103.3193, 3.0848) radius 1.5 projected
  circle A2 centre (-68.971, -6.9325) radius 1.5 projected
  circle A3 centre (-64.3204, -94.5406) radius 1.5 projected
  circle A4 centre (-97.0717, -108.9456) radius 1.5 projected
  circle A5 centre (-116.3572, -106.7764) radius 1.5 projected
  circle A6 centre (-80.6184, -105.0768) radius 1.5 projected
  circle A7 centre (-55.5918, -20.9907) radius 1.5 projected
  circle A8 centre (-84.0618, 0.6798) radius 1.5 projected
  circle A9 centre (-168.6885, -20.0217) radius 1.5 projected
  circle A10 centre (-101.5862, -52.8251) radius 24.5 projected
  line L0 (-143.1499, -110.2614) -> (-154.1203, -103.6491) projected
  line L1 (-133.8578, -104.0771) -> (-143.1499, -110.2614) projected
  arc A11 (-131.9504, -103.9087) -> (-133.8578, -104.0771) centre (-132.7497, -105.7421) ccw projected
  line L2 (-118.2736, -109.8711) -> (-131.9504, -103.9087) projected
  arc A12 (-118.2736, -109.8711) -> (-113.2383, -111.1084) centre (-101.5862, -52.8251) ccw projected
  line L3 (-113.0479, -110.1564) -> (-113.2383, -111.1084) projected
  arc A13 (-110.7619, -108.5751) -> (-113.0479, -110.1564) centre (-111.0867, -110.5485) ccw projected
  arc A14 (-110.7619, -108.5751) -> (-102.0649, -109.3231) centre (-101.5862, -52.8251) ccw projected
  arc A15 (-100.0825, -111.2716) -> (-102.0649, -109.3231) centre (-102.0818, -111.323) ccw projected
  line L4 (-100.0481, -112.6071) -> (-100.0825, -111.2716) projected
  arc A16 (-100.0481, -112.6071) -> (-93.8077, -112.1188) centre (-101.5862, -52.8251) ccw projected
  line L5 (-82.1262, -109.3721) -> (-93.8077, -112.1188) projected
  arc A17 (-82.1262, -109.3721) -> (-76.3221, -107.0282) centre (-101.5862, -52.8251) ccw projected
  line L6 (-76.8865, -105.8173) -> (-76.3221, -107.0282) projected
  arc A18 (-75.9801, -103.1896) -> (-76.8865, -105.8173) centre (-75.0737, -104.9724) ccw projected
  arc A19 (-75.9801, -103.1896) -> (-68.5278, -98.6442) centre (-101.5862, -52.8251) ccw projected
  arc A20 (-65.7766, -99.0412) -> (-68.5278, -98.6442) centre (-67.3576, -100.2661) ccw projected
  line L7 (-65.182, -99.8086) -> (-65.7766, -99.0412) projected
  arc A21 (-65.182, -99.8086) -> (-61.2256, -96.4569) centre (-101.5862, -52.8251) ccw projected
  line L8 (-50.9384, -84.1889) -> (-61.2256, -96.4569) projected
  line L9 (-50.9384, -84.1889) -> (21.5424, -27.5848) projected
  arc A22 (21.5424, -27.5848) -> (23.1865, -26.2181) centre (0, 0) ccw projected
  arc A23 (25.6192, -26.0511) -> (23.1865, -26.2181) centre (24.5114, -27.7163) ccw projected
  line L10 (25.6192, -26.0511) -> (27.0682, -27.015) projected
  line L11 (27.0682, -27.015) -> (35.3764, -14.5261) projected
  line L12 (35.3764, -14.5261) -> (33.9274, -13.5621) projected
  arc A24 (33.1414, -11.2539) -> (33.9274, -13.5621) centre (35.0352, -11.8969) ccw projected
  arc A25 (33.1414, -11.2539) -> (34.2988, 6.971) centre (0, 0) ccw projected
  arc A26 (35.3705, 9.1613) -> (34.2988, 6.971) centre (36.2587, 7.3694) ccw projected
  line L13 (35.3705, 9.1613) -> (36.9298, 9.9342) projected
  line L14 (36.9298, 9.9342) -> (30.2682, 23.3738) projected
  line L15 (30.2682, 23.3738) -> (28.7089, 22.6009) projected
  arc A27 (26.3168, 23.0743) -> (28.7089, 22.6009) centre (27.8206, 24.3929) ccw projected
  arc A28 (26.3168, 23.0743) -> (11.1123, 33.1891) centre (0, 0) ccw projected
  arc A29 (9.7513, 35.2124) -> (11.1123, 33.1891) centre (11.7473, 35.0856) ccw projected
  line L16 (9.7513, 35.2124) -> (9.8616, 36.9493) projected
  line L17 (9.8616, 36.9493) -> (-5.1082, 37.8999) projected
  line L18 (-5.1082, 37.8999) -> (-5.2185, 36.1631) projected
  arc A30 (-6.8246, 34.3282) -> (-5.2185, 36.1631) centre (-7.2145, 36.2898) ccw projected
  arc A31 (-6.8246, 34.3282) -> (-9.6196, 33.6521) centre (0, 0) ccw projected
  line L19 (-9.6196, 33.6521) -> (-104.4582, 6.5421) projected
  line L20 (-120.2244, 3.7567) -> (-104.4582, 6.5421) projected
  line L21 (-118.6463, -1.0341) -> (-120.2244, 3.7567) projected
  arc A32 (-119.947, -3.5681) -> (-118.6463, -1.0341) centre (-120.5459, -1.6599) ccw projected
  line L22 (-163.5618, -17.2551) -> (-119.947, -3.5681) projected
  arc A33 (-164.5686, -17.3049) -> (-163.5618, -17.2551) centre (-164.1607, -15.3469) ccw projected
  line L23 (-171.8906, -15.7795) -> (-164.5686, -17.3049) projected
  line L24 (-172.3553, -18.0103) -> (-171.8906, -15.7795) projected
  arc A34 (-174.021, -19.5809) -> (-172.3553, -18.0103) centre (-174.3133, -17.6024) ccw projected
  arc A35 (-174.021, -19.5809) -> (-192.9877, -32.0075) centre (-170.0752, -46.291) ccw projected
  arc A36 (-195.0928, -32.9074) -> (-192.9877, -32.0075) centre (-194.6849, -30.9495) ccw projected
  line L25 (-197.3236, -32.4427) -> (-195.0928, -32.9074) projected
  line L26 (-202.1152, -55.4432) -> (-197.3236, -32.4427) projected
  line L27 (-202.1152, -55.4432) -> (-193.8622, -57.1625) projected
  arc A37 (-154.1203, -103.6491) -> (-193.8622, -57.1625) centre (-204.0596, -106.1116) ccw projected
  circle A38 centre (-170.0752, -46.291) radius 8 projected
  circle A39 centre (-150.1212, -98.3082) radius 2.1 projected
  circle A40 centre (-192.9444, -52.7571) radius 2.1 projected
  circle A41 centre (-157.6232, -77.5824) radius 2.1 projected
  circle A42 centre (-172.7208, -61.5232) radius 2.1 projected
  line L28 (-185.1226, -43.1563) -> (-188.5725, -42.4375) projected
  arc A43 (-190.0688, -39.8678) -> (-188.5725, -42.4375) centre (-188.1646, -40.4796) ccw projected
  arc A44 (-178.7085, -27.1477) -> (-190.0688, -39.8678) centre (-170.0752, -46.291) ccw projected
  arc A45 (-175.9866, -28.3451) -> (-178.7085, -27.1477) centre (-177.8862, -28.9709) ccw projected
  line L29 (-175.9866, -28.3451) -> (-174.8841, -31.6922) projected
  arc A46 (-175.9181, -34.121) -> (-174.8841, -31.6922) centre (-176.7837, -32.318) ccw projected
  arc A47 (-175.9181, -34.121) -> (-182.8257, -41.8554) centre (-170.0752, -46.291) ccw projected
  arc A48 (-185.1226, -43.1563) -> (-182.8257, -41.8554) centre (-184.7147, -41.1983) ccw projected
  arc A49 (-151.8275, -24.8597) -> (-156.6979, -36.4255) centre (-101.5862, -52.8251) ccw projected
  arc A50 (-160.0936, -37.2016) -> (-156.6979, -36.4255) centre (-158.6148, -35.855) ccw projected
  arc A51 (-160.0936, -37.2016) -> (-165.7696, -33.4961) centre (-170.0752, -46.291) ccw projected
  arc A52 (-166.242, -29.937) -> (-165.7696, -33.4961) centre (-165.1317, -31.6005) ccw projected
  line L30 (-166.242, -29.937) -> (-154.6853, -22.2235) projected
  arc A53 (-151.8275, -24.8597) -> (-154.6853, -22.2235) centre (-153.575, -23.887) ccw projected
  arc A54 (-160.689, -66.8529) -> (-165.4906, -62.1266) centre (-204.0596, -106.1116) ccw projected
  arc A55 (-164.9337, -58.7736) -> (-165.4906, -62.1266) centre (-164.172, -60.6229) ccw projected
  arc A56 (-164.9337, -58.7736) -> (-161.5854, -56.7874) centre (-170.0752, -46.291) ccw projected
  arc A57 (-158.3364, -58.1554) -> (-161.5854, -56.7874) centre (-160.3277, -58.3424) ccw projected
  arc A58 (-158.3364, -58.1554) -> (-157.2531, -65.0807) centre (-101.5862, -52.8251) ccw projected
  arc A59 (-160.689, -66.8529) -> (-157.2531, -65.0807) centre (-159.2063, -65.5108) ccw projected
  circle A60 centre (-43.6807, 16.7845) radius 2 projected
  circle A61 centre (-12.9414, -45.3106) radius 2 projected
  circle A62 centre (-29.7575, 22.3653) radius 2 projected
  circle A63 centre (-0.1675, -37.4475) radius 2 projected
  circle A64 centre (2.1232, 33.4327) radius 1.5 projected
  circle A65 centre (27.8919, -18.555) radius 1.5 projected
  circle A66 centre (30.0151, 14.8776) radius 1.5 projected
  circle A67 centre (-46.357, -24.1058) radius 2.05 projected
  circle A68 centre (-29.3579, -24.2832) radius 2.05 projected
  circle A69 centre (-36.7396, -10.0877) radius 2.05 projected
  line L31 (-148.9024, -46.4081) -> (-136.5102, -48.7551) projected
  arc A70 (-134.07, -51.7976) -> (-136.5102, -48.7551) centre (-137.0685, -51.7027) ccw projected
  arc A71 (-134.07, -51.7976) -> (-133.8489, -56.7452) centre (-101.5862, -52.8251) ccw projected
  arc A72 (-136.2148, -60.0439) -> (-133.8489, -56.7452) centre (-136.827, -57.1071) ccw projected
  line L32 (-136.2148, -60.0439) -> (-148.4842, -62.6017) projected
  arc A73 (-152.0658, -60.0923) -> (-148.4842, -62.6017) centre (-149.0964, -59.6648) ccw projected
  arc A74 (-152.4528, -49.1389) -> (-152.0658, -60.0923) centre (-101.5862, -52.8251) ccw projected
  arc A75 (-148.9024, -46.4081) -> (-152.4528, -49.1389) centre (-149.4607, -49.3557) ccw projected
  line L33 (-141.6611, -26.5763) -> (-131.1768, -33.4435) projected
  arc A76 (-130.181, -37.3789) -> (-131.1768, -33.4435) centre (-132.8205, -35.9531) ccw projected
  arc A77 (-130.181, -37.3789) -> (-132.196, -41.9031) centre (-101.5862, -52.8251) ccw projected
  arc A78 (-135.5798, -43.8425) -> (-132.196, -41.9031) centre (-135.0215, -40.8949) ccw projected
  line L34 (-135.5798, -43.8425) -> (-147.972, -41.4954) projected
  arc A79 (-150.2779, -37.6555) -> (-147.972, -41.4954) centre (-147.4137, -38.5478) ccw projected
  arc A80 (-145.9123, -27.6022) -> (-150.2779, -37.6555) centre (-101.5862, -52.8251) ccw projected
  arc A81 (-141.6611, -26.5763) -> (-145.9123, -27.6022) centre (-143.3049, -29.0859) ccw projected
  line L35 (-118.1906, -12.9184) -> (-115.5235, -20.5451) projected
  arc A82 (-116.9382, -24.1796) -> (-115.5235, -20.5451) centre (-118.3553, -21.5354) ccw projected
  arc A83 (-116.9382, -24.1796) -> (-121.1125, -26.8448) centre (-101.5862, -52.8251) ccw projected
  arc A84 (-125.1522, -26.4453) -> (-121.1125, -26.8448) centre (-122.9149, -24.4467) ccw projected
  line L36 (-125.1522, -26.4453) -> (-130.4975, -20.4618) projected
  arc A85 (-130.0998, -16.0933) -> (-130.4975, -20.4618) centre (-128.2602, -18.4631) ccw projected
  arc A86 (-122.3629, -11.2249) -> (-130.0998, -16.0933) centre (-101.5862, -52.8251) ccw projected
  arc A87 (-118.1906, -12.9184) -> (-122.3629, -11.2249) centre (-121.0224, -13.9088) ccw projected
  line L37 (-99.1452, -9.4974) -> (-99.5965, -17.5081) projected
  arc A88 (-102.5068, -20.3382) -> (-99.5965, -17.5081) centre (-102.5918, -17.3394) ccw projected
  arc A89 (-102.5068, -20.3382) -> (-107.4323, -20.8552) centre (-101.5862, -52.8251) ccw projected
  arc A90 (-110.8038, -18.8945) -> (-107.4323, -20.8552) centre (-107.9719, -17.9042) ccw projected
  line L38 (-110.8038, -18.8945) -> (-113.4709, -11.2679) projected
  arc A91 (-111.2634, -7.3432) -> (-113.4709, -11.2679) centre (-110.6391, -10.2776) ccw projected
  arc A92 (-102.1787, -6.3289) -> (-111.2634, -7.3432) centre (-101.5862, -52.8251) ccw projected
  arc A93 (-99.1452, -9.4974) -> (-102.1787, -6.3289) centre (-102.1405, -9.3287) ccw projected
  line L39 (-72.3708, -15.0566) -> (-80.5995, -24.6151) projected
  arc A94 (-84.4544, -25.2071) -> (-80.5995, -24.6151) centre (-82.873, -22.6578) ccw projected
  arc A95 (-84.4544, -25.2071) -> (-88.8497, -22.9247) centre (-101.5862, -52.8251) ccw projected
  arc A96 (-90.5236, -19.2265) -> (-88.8497, -22.9247) centre (-87.6741, -20.1647) ccw projected
  line L40 (-90.5236, -19.2265) -> (-86.604, -7.322) projected
  arc A97 (-82.64, -5.4749) -> (-86.604, -7.322) centre (-83.7544, -8.2602) ccw projected
  arc A98 (-72.9605, -10.6165) -> (-82.64, -5.4749) centre (-101.5862, -52.8251) ccw projected
  arc A99 (-72.3708, -15.0566) -> (-72.9605, -10.6165) centre (-74.6444, -13.0993) ccw projected
  line L41 (-58.8166, -31.2436) -> (-70.0059, -36.8897) projected
  arc A100 (-73.912, -35.7844) -> (-70.0059, -36.8897) centre (-71.3574, -34.2114) ccw projected
  arc A101 (-73.912, -35.7844) -> (-76.8225, -31.7773) centre (-101.5862, -52.8251) ccw projected
  arc A102 (-76.8102, -27.8772) -> (-76.8225, -31.7773) centre (-74.5366, -29.8344) ccw projected
  line L42 (-76.8102, -27.8772) -> (-68.5815, -18.3187) projected
  arc A103 (-64.1031, -18.2417) -> (-68.5815, -18.3187) centre (-66.308, -20.276) ccw projected
  arc A104 (-57.5795, -27.049) -> (-64.1031, -18.2417) centre (-101.5862, -52.8251) ccw projected
  arc A105 (-58.8166, -31.2436) -> (-57.5795, -27.049) centre (-60.1681, -28.5653) ccw projected
  line L43 (-58.7238, -58.3986) -> (-66.6622, -56.8951) projected
  arc A106 (-69.1024, -53.8527) -> (-66.6622, -56.8951) centre (-66.1039, -53.9475) ccw projected
  arc A107 (-69.1024, -53.8527) -> (-69.3235, -48.905) centre (-101.5862, -52.8251) ccw projected
  arc A108 (-66.9576, -45.6063) -> (-69.3235, -48.905) centre (-66.3454, -48.5432) ccw projected
  line L44 (-66.9576, -45.6063) -> (-59.1031, -43.9689) projected
  arc A109 (-55.5187, -46.4975) -> (-59.1031, -43.9689) centre (-58.4908, -46.9058) ccw projected
  arc A110 (-55.171, -55.6321) -> (-55.5187, -46.4975) centre (-101.5862, -52.8251) ccw projected
  arc A111 (-58.7238, -58.3986) -> (-55.171, -55.6321) centre (-58.1655, -55.451) ccw projected
  line L45 (-65.2838, -76.603) -> (-71.9956, -72.2068) projected
  arc A112 (-72.9914, -68.2714) -> (-71.9956, -72.2068) centre (-70.3519, -69.6972) ccw projected
  arc A113 (-72.9914, -68.2714) -> (-70.9764, -63.7472) centre (-101.5862, -52.8251) ccw projected
  arc A114 (-67.5926, -61.8078) -> (-70.9764, -63.7472) centre (-68.1509, -64.7554) ccw projected
  line L46 (-67.5926, -61.8078) -> (-59.6542, -63.3113) projected
  arc A115 (-57.3591, -67.1854) -> (-59.6542, -63.3113) centre (-60.2125, -66.2589) ccw projected
  arc A116 (-61.023, -75.5601) -> (-57.3591, -67.1854) centre (-101.5862, -52.8251) ccw projected
  arc A117 (-65.2838, -76.603) -> (-61.023, -75.5601) centre (-63.64, -74.0934) ccw projected
  line L47 (-83.4854, -97.0107) -> (-87.6489, -85.1052) projected
  arc A118 (-86.2342, -81.4707) -> (-87.6489, -85.1052) centre (-84.8171, -84.1149) ccw projected
  arc A119 (-86.2342, -81.4707) -> (-82.0599, -78.8054) centre (-101.5862, -52.8251) ccw projected
  arc A120 (-78.0202, -79.2049) -> (-82.0599, -78.8054) centre (-80.2575, -81.2036) ccw projected
  line L48 (-78.0202, -79.2049) -> (-69.6705, -88.5517) projected
  arc A121 (-70.0529, -92.9081) -> (-69.6705, -88.5517) centre (-71.9078, -90.5503) ccw projected
  arc A122 (-79.3453, -98.72) -> (-70.0529, -92.9081) centre (-101.5862, -52.8251) ccw projected
  arc A123 (-83.4854, -97.0107) -> (-79.3453, -98.72) centre (-80.6536, -96.0203) ccw projected
  line L49 (-104.2809, -100.6554) -> (-103.5759, -88.1421) projected
  arc A124 (-100.6656, -85.3121) -> (-103.5759, -88.1421) centre (-100.5806, -88.3109) ccw projected
  arc A125 (-100.6656, -85.3121) -> (-95.7401, -84.795) centre (-101.5862, -52.8251) ccw projected
  arc A126 (-92.3686, -86.7557) -> (-95.7401, -84.795) centre (-95.2005, -87.7461) ccw projected
  line L50 (-92.3686, -86.7557) -> (-88.2051, -98.6612) projected
  arc A127 (-90.3776, -102.5782) -> (-88.2051, -98.6612) centre (-91.0369, -99.6515) ccw projected
  arc A128 (-101.2668, -103.8241) -> (-90.3776, -102.5782) centre (-101.5862, -52.8251) ccw projected
  arc A129 (-104.2809, -100.6554) -> (-101.2668, -103.8241) centre (-101.2856, -100.8242) ccw projected
  line L51 (-130.8016, -90.5936) -> (-122.5729, -81.0352) projected
  arc A130 (-118.718, -80.4431) -> (-122.5729, -81.0352) centre (-120.2993, -82.9925) ccw projected
  arc A131 (-118.718, -80.4431) -> (-114.3227, -82.7255) centre (-101.5862, -52.8251) ccw projected
  arc A132 (-112.6488, -86.4238) -> (-114.3227, -82.7255) centre (-115.4983, -85.4855) ccw projected
  line L52 (-112.6488, -86.4238) -> (-116.5684, -98.3282) projected
  arc A133 (-120.5324, -100.1753) -> (-116.5684, -98.3282) centre (-119.418, -97.39) ccw projected
  arc A134 (-130.2119, -95.0338) -> (-120.5324, -100.1753) centre (-101.5862, -52.8251) ccw projected
  arc A135 (-130.8016, -90.5936) -> (-130.2119, -95.0338) centre (-128.528, -92.5509) ccw projected
  circle A136 centre (-143.2853, -74.5088) radius 2.05 projected
  circle A137 centre (-129.9771, -67.5885) radius 2.05 projected
  line L53 (-50.3266, -9.3898) -> (-50.2576, 7.0148) projected
  arc A138 (-48.8073, 8.9294) -> (-50.2576, 7.0148) centre (-48.2576, 7.0064) ccw projected
  line L54 (-48.8073, 8.9294) -> (-35.9765, 12.5971) projected
  arc A139 (-33.5119, 10.0972) -> (-35.9765, 12.5971) centre (-35.4269, 10.6742) ccw projected
  arc A140 (-33.5119, 10.0972) -> (-34.8805, 2.8895) centre (0, 0) ccw projected
  arc A141 (-37.5189, -2.412) -> (-34.8805, 2.8895) centre (-42.8532, 3.55) ccw projected
  line L55 (-37.5189, -2.412) -> (-46.993, -10.8887) projected
  arc A142 (-50.3266, -9.3898) -> (-46.993, -10.8887) centre (-48.3266, -9.3983) ccw projected
  line L56 (-22.1863, -44.6489) -> (-35.0333, -35.1325) projected
  arc A143 (-33.7812, -31.5263) -> (-35.0333, -35.1325) centre (-33.8429, -33.5254) ccw projected
  line L57 (-33.7812, -31.5263) -> (-9.7002, -32.2696) projected
  arc A144 (-8.5309, -35.8449) -> (-9.7002, -32.2696) centre (-9.7619, -34.2687) ccw projected
  line L58 (-8.5309, -35.8449) -> (-19.7649, -44.6181) projected
  arc A145 (-22.1863, -44.6489) -> (-19.7649, -44.6181) centre (-20.9959, -43.0418) ccw projected
  arc A146 (-58.7261, -9.42) -> (-70.0175, -0.6292) centre (-101.5862, -52.8251) ccw projected
  arc A147 (-69.5321, 3.0051) -> (-70.0175, -0.6292) centre (-68.9824, 1.0822) ccw projected
  line L59 (-69.5321, 3.0051) -> (-57.8182, 6.3536) projected
  arc A148 (-55.2686, 4.4222) -> (-57.8182, 6.3536) centre (-57.2686, 4.4306) ccw projected
  line L60 (-55.2686, 4.4222) -> (-55.3208, -8.0052) projected
  arc A149 (-58.7261, -9.42) -> (-55.3208, -8.0052) centre (-57.3208, -7.9968) ccw projected
  line L61 (-27.1252, -50.3662) -> (-37.4859, -58.4574) projected
  arc A150 (-40.7128, -56.7524) -> (-37.4859, -58.4574) centre (-38.7169, -56.8811) ccw projected
  arc A151 (-40.7128, -56.7524) -> (-41.8084, -40.6753) centre (-101.5862, -52.8251) ccw projected
  arc A152 (-38.658, -38.6698) -> (-41.8084, -40.6753) centre (-39.8485, -40.2769) ccw projected
  line L62 (-38.658, -38.6698) -> (-27.1657, -47.1828) projected
  arc A153 (-27.1252, -50.3662) -> (-27.1657, -47.1828) centre (-28.3562, -48.7899) ccw projected
  arc A154 (3.578, 22.065) -> (-0.4133, 22.2565) centre (1.5867, 22.2515) ccw projected
  arc A155 (22.512, 1.2224) -> (3.578, 22.065) centre (0.5323, 0.2768) ccw projected
  arc A156 (22.3205, -2.7688) -> (22.512, 1.2224) centre (22.507, -0.7775) ccw projected
  arc A157 (1.478, -21.7029) -> (22.3205, -2.7688) centre (0.5323, 0.2768) ccw projected
  arc A158 (-2.5133, -21.5114) -> (1.478, -21.7029) centre (-0.522, -21.6979) ccw projected
  arc A159 (-21.4473, -0.6688) -> (-2.5133, -21.5114) centre (0.5323, 0.2768) ccw projected
  arc A160 (-21.2558, 3.3225) -> (-21.4473, -0.6688) centre (-21.4424, 1.3312) ccw projected
  arc A161 (-0.4133, 22.2565) -> (-21.2558, 3.3225) centre (0.5323, 0.2768) ccw projected
  line L63 (0.5323, 0.2768) -> (0, 0)
  circle A162 centre (0.5323, 0.2768) radius 22
  line L64 (-0.522, -21.6979) -> (-21.4424, 1.3312)
  line L65 (0.5323, 0.2768) -> (-15.7517, -14.5161)
  circle A163 centre (-15.7517, -14.5161) radius 2
  circle A164 centre (15.3253, -16.0072) radius 2
  circle A165 centre (16.8163, 15.0697) radius 2
  circle A166 centre (-14.2606, 16.5608) radius 2
  point P0 (0, 0)
  point P1 (-14.341, -15.9338)
  point P2 (1.478, -21.7029)
  point P3 (13.7853, -17.2833)
  point P4 (16.743, -14.5965)
  point P5 (22.512, 1.2224)
  point P6 (18.0925, 13.5298)
  point P7 (15.4056, 16.4874)
  point P8 (-0.4133, 22.2565)
  point P9 (-12.7206, 17.837)
  point P10 (-15.6783, 15.1501)
  point P11 (-21.4473, -0.6688)
  point P12 (-17.0278, -12.9762)
  dimension "d64" = 44
  dimension "d65" = 4
  dimension "d68" = 360
  constraints: 6 end point, 4 centre point, 2 coincident, 1 perpendicular, 12 other
  measures "d65" diameter of A163
extrude "Extrusion12" cut sketch "Sketch13" against normal blind 10 contours A155 A165 A162 A157 A164 L64 A161 A166 | A165 A155 | A155 A165 | A166 A161 | A161 A166 | A162 L64 L65 A163 A159 | A164 A157 | A157 A164 | A163 L65 A159 | A159 A163 | L64 A162 A159 A163 L65 | L65 A163 A159
sketch "Sketch14" plane through (0, 0, 0) normal (0, 0, 1) x (1, 0, 0)
  circle A0 centre (2.1232, 33.4327) radius 1.5 projected
  circle A1 centre (30.0151, 14.8776) radius 1.5 projected
  circle A2 centre (27.8919, -18.555) radius 1.5 projected
  line L0 (0, 0) -> (27.8919, -18.555)
  line L1 (0, 0) -> (30.0151, 14.8776)
  line L2 (0, 0) -> (2.1232, 33.4327)
  line L3 (-5.6153, 29.916) -> (-5.1082, 37.8999)
  line L4 (-5.1082, 37.8999) -> (9.8616, 36.9493)
  line L5 (9.8616, 36.9493) -> (9.3546, 28.9654)
  line L6 (9.3546, 28.9654) -> (-5.6153, 29.916)
  line L7 (-5.6153, 29.916) -> (9.8616, 36.9493) construction
  line L8 (-5.1082, 37.8999) -> (9.3546, 28.9654) construction
  line L9 (36.9298, 9.9342) -> (29.762, 6.3814)
  line L10 (29.762, 6.3814) -> (23.1004, 19.821)
  line L11 (23.1004, 19.821) -> (30.2682, 23.3738)
  line L12 (30.2682, 23.3738) -> (36.9298, 9.9342)
  line L13 (36.9298, 9.9342) -> (23.1004, 19.821) construction
  line L14 (29.762, 6.3814) -> (30.2682, 23.3738) construction
  line L15 (27.0682, -27.015) -> (20.4074, -22.584)
  line L16 (20.4074, -22.584) -> (28.7157, -10.095)
  line L17 (28.7157, -10.095) -> (35.3764, -14.5261)
  line L18 (35.3764, -14.5261) -> (27.0682, -27.015)
  line L19 (27.0682, -27.015) -> (28.7157, -10.095) construction
  line L20 (20.4074, -22.584) -> (35.3764, -14.5261) construction
  arc A3 (0.3834, -34.7229) -> (-12.1292, 32.9063) centre (0.5323, 0.2768) ccw projected
  point P0 (32.9518, -12.9131)
  point P1 (24.4517, -25.2744)
  point P2 (27.8396, 22.1701)
  point P3 (34.4966, 8.7282)
  point P4 (-5.306, 34.7864)
  point P5 (9.6782, 34.0607)
  dimension "d72" = 8
  dimension "d73" = 15
  dimension "d74" = 8
  dimension "d75" = 15
  dimension "d76" = 8
  dimension "d77" = 15
  constraints: 42 end point, 6 midpoint, 6 parallel, 6 perpendicular
  measures "d72" distance of L3.start L3.end
  measures "d73" distance of L3.end L4.end
  measures "d74" distance of L9.start L9.end
  measures "d75" distance of L9.end L10.end
  measures "d76" distance of L15.start L15.end
  measures "d77" distance of L15.end L16.end
extrude "Extrusion13" add sketch "Sketch14" against normal blind 5 contours A3 L17 L18 L15 | A3 L11 L12 L9 | A3 L3 L4 L5
fillet "Fillet5" radius 2 6 edges at (24.4517, -25.2744, -2.5) (32.9518, -12.9131, -2.5) (34.4966, 8.7282, -2.5) (27.8396, 22.1701, -2.5) (9.6782, 34.0607, -2.5) (-5.306, 34.7864, -2.5)
body "Solid1"
